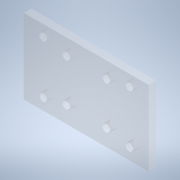
# Autodesk Inventor part: interplate
Saved by Autodesk Inventor 2021 (Build 250183000, 183)
## iProperties
Created: 2023-10-29
Part Number: interplate
Material: PMMA Plastic
Document SubType Name: Modeling
Designer: M
Density: 1.23835 g/cm^3
Appearance: Polycarbonate - Clear
Mass: 42.9 g
Surface Area: 143.724 cm^2
Volume: 34.6428 cm^3
Author: M
Autodesk Inventor part; units mm, degrees
ref_plane "YZ Plane" through (0, 0, 0) normal (1, 0, 0) x (0, 1, 0)
ref_plane "XZ Plane" through (0, 0, 0) normal (0, 1, 0) x (-1, 0, 0)
ref_plane "XY Plane" through (0, 0, 0) normal (0, 0, 1) x (1, 0, 0)
sketch "Sketch1" plane through (0, 0, 0) normal (0, 0, 1) x (1, 0, 0)
  line L0 (0, 0) -> (-100, 0)
  line L1 (-100, 0) -> (-100, -60)
  line L2 (-100, -60) -> (0, -60)
  line L3 (0, -60) -> (0, 0)
  circle A0 centre (-15.5, -9) radius 3
  circle A1 centre (-15.5, -51) radius 3
  circle A2 centre (-34, -47) radius 3
  circle A3 centre (-66, -47) radius 3
  circle A4 centre (-34, -13) radius 3
  circle A5 centre (-66, -13) radius 3
  circle A6 centre (-84.5, -9) radius 3
  circle A7 centre (-84.5, -51) radius 3
  line L4 (-66, -47) -> (-66, -13)
  line L5 (-66, -13) -> (-34, -13)
  line L6 (-34, -13) -> (-34, -47)
  line L7 (-34, -47) -> (-66, -47)
  line L8 (-84.5, -51) -> (-84.5, -9)
  line L9 (-15.5, -51) -> (-15.5, -9)
  line L10 (-15.5, -51) -> (-84.5, -51)
  line L11 (-84.5, -9) -> (-15.5, -9)
  dimension "d0" = 100
  dimension "d1" = 60
  dimension "d4" = 6
  dimension "d5" = 6
  dimension "d6" = 6
  dimension "d7" = 6
  dimension "d8" = 34
  dimension "d9" = 32
  dimension "d10" = 13
  dimension "d11" = 34
  dimension "d12" = 6
  dimension "d13" = 6
  dimension "d14" = 6
  dimension "d15" = 6
  dimension "d16" = 42
  dimension "d17" = 69
  dimension "d18" = 9
  dimension "d19" = 15.5
  constraints: 24 end point, 8 centre point, 4 parallel, 3 horizontal, 3 perpendicular, 2 vertical, 1 coincident, 1 other
  measures "d0" distance of L2.end L1.end
  measures "d1" distance of L1.end L0.end
  measures "d4" diameter of A2
  measures "d5" diameter of A3
  measures "d6" diameter of A5
  measures "d7" diameter of A4
  measures "d8" distance of L4.start L4.end
  measures "d9" distance of L4.end L5.end
  measures "d10" distance between parallel lines of L2 L7
  measures "d11" distance between parallel lines of L3 L6
  measures "d12" diameter of A6
  measures "d13" diameter of A7
  measures "d14" diameter of A0
  measures "d15" diameter of A1
  measures "d16" distance of L8.start L8.end
  measures "d17" distance of L8.end L9.end
  measures "d18" distance between parallel lines of L2 L10
  measures "d19" distance between parallel lines of L3 L9
extrude "Extrusion1" add sketch "Sketch1" along normal blind 6 contours L3 L2 L1 L0 | A0 L9 A1 L10 A7 L8 A6 L11 | A2 L7 A3 L4 A5 L5 A4 L6
equation "\"d5\" = d4"
equation "\"d6\" = d4"
equation "\"d7\" = d4"
equation "\"d10\" = -0.5 * d8 + 0.5 * d1"
equation "\"d11\" = -0.5 * d9 + 0.5 * d0"
equation "\"d13\" = d12"
equation "\"d14\" = d12"
equation "\"d15\" = d12"
equation "\"d18\" = -0.5 * d16 + 0.5 * d1"
equation "\"d19\" = -0.5 * d17 + 0.5 * d0"
body "Solid1"
